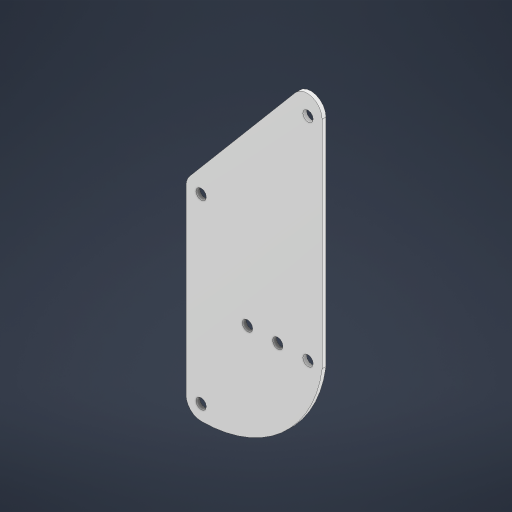
# Autodesk Inventor part: sled
Saved by Autodesk Inventor 2024 (Build 280153000, 153)
## iProperties
Created: 2023-10-18
Part Number: sled
Material: Acetal Resin, White
Document SubType Name: Sheet Metal
Designer: Averey Ku
Density: 1.425 g/cm^3
Appearance: Smooth - White
Flat Pattern Width: 14.1545 cm
Flat Pattern Length: 5.715 cm
Flat Pattern Area: 80.893 cm^2
Sheet Metal Rule: Default_mm
Sheet Metal Width: 5.573 in
Sheet Metal Length: 2.250 in
Sheet Metal Area: 12.538 in^2
Author: Averey Ku
Autodesk Inventor part; units mm, degrees
ref_plane "YZ Plane" through (0, 0, 0) normal (1, 0, 0) x (0, 1, 0)
ref_plane "XZ Plane" through (0, 0, 0) normal (0, 1, 0) x (-1, 0, 0)
ref_plane "XY Plane" through (0, 0, 0) normal (0, 0, 1) x (1, 0, 0)
sketch "Sketch1" plane through (0, 0, 0) normal (0, 0, 1) x (1, 0, 0)
  circle A0 centre (-26.6729, -59.6511) radius 2.1844
  circle A1 centre (-26.6729, 16.5489) radius 2.1844
  circle A2 centre (-7.2038, -21.5511) radius 2.1844
  circle A3 centre (5.4962, -21.5511) radius 2.1844
  arc A4 (-31.5248, 20.6455) -> (-33.0229, 16.5489) centre (-26.6729, 16.5489) ccw
  arc A5 (-33.0229, -59.6511) -> (-26.6706, -66.0011) centre (-26.6729, -59.6511) ccw
  arc A6 (-26.6706, -66.0011) -> (24.1271, -21.5511) centre (-26.689, -14.7292) ccw
  line L0 (-31.5248, 20.6455) -> (12.9252, 73.2906)
  line L1 (15.1232, 75.8938) -> (-31.5248, 20.6455)
  line L2 (12.9252, 73.2906) -> (-31.5248, 20.6455)
  line L3 (24.1271, -21.5511) -> (24.1271, 69.194)
  circle A7 centre (18.1962, -21.5511) radius 2.1844
  circle A8 centre (18.1962, 67.3489) radius 2.1844
  arc A9 (24.1271, 69.194) -> (12.9252, 73.2906) centre (17.7771, 69.194) ccw
  line L4 (-33.0229, -59.6511) -> (-33.0229, 16.5489)
  dimension "d6" = 12.7
  dimension "d7" = 12.7
  dimension "d9" = 4.3688
  dimension "d10" = 4.3688
  dimension "d11" = 6.35
  constraints: 10 centre point, 10 end point, 8 point on circle, 8 tangent, 2 coincident, 1 vertical
  measures "d6" diameter of A4
  measures "d7" diameter of A5
  measures "d9" diameter of A7
  measures "d10" diameter of A8
  measures "d11" radius of A9
extrude "Extrusion1" add sketch "Sketch1" along normal blind 1.5875
equation "\"BendRadius\" = Thickness"
equation "\"BendReliefWidth\" = Thickness"
equation "\"BendReliefDepth\" = 0.5 * Thickness"
equation "\"CornerReliefSize\" = 4 * Thickness"
equation "\"MinimumRemnant\" = 2 * Thickness"
equation "\"TransitionRadius\" = BendRadius"
equation "\"JacobiRadiusSize\" = BendRadius"
equation "\"GapSize\" = Thickness"
equation "\"Thickness\" = 1.5875"
body "Solid1"
